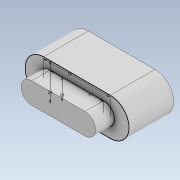
# Autodesk Inventor part: Gabel_DistanzStopper
Saved by Autodesk Inventor 2022 (Build 260153000, 153)
## iProperties
Created: 2022-10-13
Part Number: Gabel_DistanzStopper
Material: Generisch
Document SubType Name: Modeling
Designer: alexw
Density: 1 g/cm^3
Appearance: Vorgabe
Height: 47,623 mm
Author: alexw
Autodesk Inventor part; units mm, degrees
ref_plane "YZ Plane" through (0, 0, 0) normal (1, 0, 0) x (0, 1, 0)
ref_plane "XZ Plane" through (0, 0, 0) normal (0, 1, 0) x (-1, 0, 0)
ref_plane "XY Plane" through (0, 0, 0) normal (0, 0, 1) x (1, 0, 0)
sketch "Skizze1" plane through (0, 0, 0) normal (0, 0, 1) x (1, 0, 0)
  line L0 (-20, 0) -> (20, 0) construction
  line L1 (-20, -8) -> (20, -8)
  line L2 (20, 8) -> (-20, 8)
  arc A0 (-20, 8) -> (-20, -8) centre (-20, 0) ccw
  arc A1 (20, -8) -> (20, 8) centre (20, 0) ccw
  line L3 (-25, 0) -> (25, 0) construction
  line L4 (-25, -14) -> (25, -14)
  line L5 (25, 14) -> (-25, 14)
  arc A2 (-25, 14) -> (-25, -14) centre (-25, 0) ccw
  arc A3 (25, -14) -> (25, 14) centre (25, 0) ccw
  point P0 (0, 0)
  dimension "d0" = 16
  dimension "d1" = 40
  dimension "d2" = 28
  dimension "d3" = 50
  constraints: 16 end point, 8 point on circle, 8 tangent, 4 centre point, 2 horizontal, 2 midpoint, 2 parallel
  measures "d0" distance between parallel lines of L1 L2
  measures "d1" distance of L0.end L0.start
  measures "d2" distance between parallel lines of L4 L5
  measures "d3" distance of L3.start L3.end
extrude "Extrusion1" add sketch "Skizze1" along normal blind 14 contours A0 L2 A1 L1
extrude "Extrusion2" add sketch "Skizze1" against normal blind 33.623 contours A0 L2 A1 L1 | A2 L5 A3 L4
equation "\"Height\" = 47.623"
